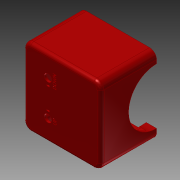
# Autodesk Inventor part: Durometer_Electronics_Enclosure_Lid
Saved by Autodesk Inventor 2015 (Build 190159000, 159)
## iProperties
Created: 2015-01-04
Part Number: Durometer_Electronics_Enclosure_Lid
Material: Generic
Document SubType Name: Modeling
Designer: Drew
Density: 1 g/cm^3
Appearance: Smooth - Red
Author: Drew
Autodesk Inventor part; units mm, degrees
ref_plane "YZ Plane" through (0, 0, 0) normal (1, 0, 0) x (0, 1, 0)
ref_plane "XZ Plane" through (0, 0, 0) normal (0, 1, 0) x (-1, 0, 0)
ref_plane "XY Plane" through (0, 0, 0) normal (0, 0, 1) x (1, 0, 0)
sketch "Sketch1" plane through (0, 0, 0) normal (0, 0, 1) x (1, 0, 0)
  line L0 (28.575, -34.925) -> (-28.575, -34.925)
  line L1 (-34.925, -28.575) -> (-34.925, 28.575)
  line L2 (-28.575, 34.925) -> (28.575, 34.925)
  line L3 (34.925, 28.575) -> (34.925, -28.575)
  line L4 (34.925, -34.925) -> (-34.925, 34.925) construction
  line L5 (-34.925, -34.925) -> (34.925, 34.925) construction
  arc A0 (-28.575, 34.925) -> (-34.925, 28.575) centre (-28.575, 28.575) ccw
  arc A1 (34.925, 28.575) -> (28.575, 34.925) centre (28.575, 28.575) ccw
  arc A2 (28.575, -34.925) -> (34.925, -28.575) centre (28.575, -28.575) ccw
  arc A3 (-34.925, -28.575) -> (-28.575, -34.925) centre (-28.575, -28.575) ccw
  point P0 (0, 0)
  dimension "d0" = 69.85
  dimension "d1" = 69.85
  dimension "d2" = 6.35
  constraints: 12 end point, 8 point on circle, 8 point on line, 8 tangent, 4 centre point, 3 equal radius, 2 midpoint, 2 parallel, 1 horizontal, 1 perpendicular
  measures "d0" distance of L4.end L5.end
  measures "d1" distance between parallel lines of L0 L2
  measures "d2" radius of A0
extrude "Extrusion1" add sketch "Sketch1" along normal blind 50.8
shell "Shell1" thickness 2.032 removed faces 1 at (9.525, 7.4083, 0)
sketch "Sketch4" plane through (0, 0, 0) normal (0, 0, -1) x (-1, 0, 0)
  arc A0 (-32.893, -28.575) -> (-28.575, -32.893) centre (-28.575, -28.575) ccw projected
  line L0 (-43.2886, 0) -> (36.2185, 0)
  line L1 (0, 45.1294) -> (0, -40.5019)
  line L2 (-28.575, -24.257) -> (-32.893, -24.257)
  line L3 (-24.257, -28.575) -> (-24.257, -32.893)
  line L4 (-24.257, -32.893) -> (-28.575, -32.893)
  line L5 (-32.893, -24.257) -> (-32.893, -28.575)
  arc A1 (-32.893, -28.575) -> (-28.575, -32.893) centre (-28.575, -28.575) ccw
  arc A2 (-24.257, -28.575) -> (-28.575, -24.257) centre (-28.575, -28.575) ccw
  arc A3 (-28.575, 32.893) -> (-32.893, 28.575) centre (-28.575, 28.575) ccw
  line L6 (-28.575, 24.257) -> (-32.893, 24.257)
  line L7 (-24.257, 28.575) -> (-24.257, 32.893)
  line L8 (-24.257, 32.893) -> (-28.575, 32.893)
  line L9 (-32.893, 24.257) -> (-32.893, 28.575)
  arc A4 (-28.575, 32.893) -> (-32.893, 28.575) centre (-28.575, 28.575) ccw
  arc A5 (-28.575, 24.257) -> (-24.257, 28.575) centre (-28.575, 28.575) ccw
  arc A6 (28.575, -32.893) -> (32.893, -28.575) centre (28.575, -28.575) ccw
  line L10 (28.575, -24.257) -> (32.893, -24.257)
  line L11 (24.257, -28.575) -> (24.257, -32.893)
  line L12 (24.257, -32.893) -> (28.575, -32.893)
  line L13 (32.893, -24.257) -> (32.893, -28.575)
  arc A7 (28.575, -32.893) -> (32.893, -28.575) centre (28.575, -28.575) ccw
  arc A8 (28.575, -24.257) -> (24.257, -28.575) centre (28.575, -28.575) ccw
  arc A9 (32.893, 28.575) -> (28.575, 32.893) centre (28.575, 28.575) ccw
  line L14 (28.575, 24.257) -> (32.893, 24.257)
  line L15 (24.257, 28.575) -> (24.257, 32.893)
  line L16 (24.257, 32.893) -> (28.575, 32.893)
  line L17 (32.893, 24.257) -> (32.893, 28.575)
  arc A10 (32.893, 28.575) -> (28.575, 32.893) centre (28.575, 28.575) ccw
  arc A11 (24.257, 28.575) -> (28.575, 24.257) centre (28.575, 28.575) ccw
  circle A12 centre (-28.575, -28.575) radius 1.45
  circle A13 centre (-28.575, 28.575) radius 1.45
  circle A14 centre (28.575, -28.575) radius 1.45
  circle A15 centre (28.575, 28.575) radius 1.45
  point P0 (0, 0)
  dimension "d7" = 4.318
  dimension "d8" = 4.318
  dimension "d11" = 2.9
  constraints: 36 end point, 27 symmetric about line, 22 point on circle, 15 centre point, 5 coincident, 4 tangent, 2 horizontal, 2 point on line, 1 vertical, 12 other
  measures "d7" distance of L2.end L5.end
  measures "d8" distance of L3.start L3.end
  measures "d11" diameter of A12
extrude "Extrusion2" add sketch "Sketch4" against normal up to surface (48.768 mm away)
fillet "Fillet2" radius 3.175 24 edges at (33.0651, 33.0651, 50.8) (0, 34.925, 50.8) (-33.0651, 33.0651, 50.8) (-34.925, 0, 50.8) (-33.0651, -33.0651, 50.8) (0, -34.925, 50.8) (33.0651, -33.0651, 50.8) (34.925, 0, 50.8) (32.893, 0, 48.768) (24.257, -30.734, 48.768) (30.734, -24.257, 48.768) (25.5217, -25.5217, 48.768) (0, -32.893, 48.768) (0, 32.893, 48.768) (30.734, 24.257, 48.768) (24.257, 30.734, 48.768) (25.5217, 25.5217, 48.768) (-30.734, -24.257, 48.768) (-24.257, -30.734, 48.768) (-25.5217, -25.5217, 48.768) (-32.893, 0, 48.768) (-24.257, 30.734, 48.768) (-30.734, 24.257, 48.768) (-25.5217, 25.5217, 48.768)
sketch "Sketch5" plane through (0, 0, 50.8) normal (0, 0, 1) x (1, 0, 0)
  circle A0 centre (-12.7, -15.875) radius 3.429
  line L0 (-50.1018, 0) -> (45.2159, 0)
  line L1 (-12.7, -24.1987) -> (-12.7, -7.4873)
  line L2 (-11.43, -9.144) -> (-13.97, -9.144)
  line L3 (-13.97, -9.144) -> (-13.97, -10.414)
  line L4 (-13.97, -10.414) -> (-11.43, -10.414)
  line L5 (-11.43, -10.414) -> (-11.43, -9.144)
  line L6 (-11.43, -9.144) -> (-13.97, -10.414) construction
  line L7 (-13.97, -9.144) -> (-11.43, -10.414) construction
  circle A1 centre (-12.7, 15.875) radius 3.429
  line L8 (-12.7, 24.1987) -> (-12.7, 7.4873)
  line L9 (-11.43, 9.144) -> (-13.97, 9.144)
  line L10 (-13.97, 9.144) -> (-13.97, 10.414)
  line L11 (-13.97, 10.414) -> (-11.43, 10.414)
  line L12 (-11.43, 10.414) -> (-11.43, 9.144)
  line L13 (-11.43, 9.144) -> (-13.97, 10.414) construction
  line L14 (-13.97, 9.144) -> (-11.43, 10.414) construction
  point P0 (0, 0)
  point P1 (-12.7, -9.779)
  point P2 (-12.7, 9.779)
  dimension "d31" = 6.096
  dimension "d32" = 6.858
  dimension "d33" = 2.54
  dimension "d34" = 1.27
  dimension "d35" = 31.75
  dimension "d36" = 12.7
  constraints: 30 end point, 8 symmetric about line, 4 midpoint, 3 point on line, 2 centre point, 2 horizontal, 2 parallel, 1 perpendicular, 1 vertical, 1 other
  measures "d31" distance of A0.centre point (-12.7, -9.779)
  measures "d32" diameter of A0
  measures "d33" distance of L2.start L2.end
  measures "d34" distance of L2.end L3.end
  measures "d35" diameter of A0.centre L0
  measures "d36" horizontal distance of point (0, 0) A0.centre
extrude "Extrusion3" cut sketch "Sketch5" against normal through all
sketch "Sketch6" plane through (0, 0, 50.8) normal (0, 0, 1) x (1, 0, 0)
  line L0 (-8.0796, -18.1611) -> (-8.0796, -12.998) construction
  line L1 (-8.0796, -12.998) -> (-4.9046, -12.998) construction
  line L2 (-4.9046, -12.998) -> (-4.9046, -18.1611) construction
  line L3 (-4.9046, -18.1611) -> (-8.0796, -18.1611) construction
  line L4 (-8.3173, 9.6901) -> (-8.3173, 22.3271) construction
  line L5 (-8.3173, 22.3271) -> (-5.1423, 22.3271) construction
  line L6 (-5.1423, 22.3271) -> (-5.1423, 9.6901) construction
  line L7 (-5.1423, 9.6901) -> (-8.3173, 9.6901) construction
  line L8 (-18.4562, -15.5796) -> (0.4358, -15.5796)
  line L9 (-19.415, 16.0086) -> (-0.523, 16.0086)
  spline S0 degree 2 poles (-4.9674, -16.7878) (-4.9674, -17.057) (-5.1082, -17.4572) (-5.249, -17.598) knots 0 0 0 1 2 2 2
  spline S1 degree 2 poles (-5.249, -17.598) (-5.4071, -17.7585) (-5.8517, -17.8894) (-6.1777, -17.8894) knots 0 0 0 1 2 2 2
  line L10 (-6.1777, -17.8894) -> (-8.0796, -17.8894)
  line L11 (-8.0796, -17.8894) -> (-8.0796, -17.4843)
  line L12 (-8.0796, -17.4843) -> (-6.1777, -17.4843)
  spline S2 degree 2 poles (-6.1777, -17.4843) (-5.9653, -17.4843) (-5.6788, -17.43) (-5.5627, -17.3534) knots 0 0 0 1 2 2 2
  spline S3 degree 2 poles (-5.5627, -17.3534) (-5.4392, -17.2719) (-5.3132, -16.9903) (-5.3132, -16.7878) knots 0 0 0 1 2 2 2
  spline S4 degree 2 poles (-5.3132, -16.7878) (-5.3132, -16.5976) (-5.4392, -16.3012) (-5.5627, -16.2197) knots 0 0 0 1 2 2 2
  spline S5 degree 2 poles (-5.5627, -16.2197) (-5.6788, -16.1431) (-5.9628, -16.0888) (-6.1678, -16.0888) knots 0 0 0 1 2 2 2
  line L13 (-6.1678, -16.0888) -> (-8.0796, -16.0888)
  line L14 (-8.0796, -16.0888) -> (-8.0796, -15.6837)
  line L15 (-8.0796, -15.6837) -> (-6.1777, -15.6837)
  spline S6 degree 2 poles (-6.1777, -15.6837) (-5.8591, -15.6837) (-5.4046, -15.8121) (-5.249, -15.9752) knots 0 0 0 1 2 2 2
  spline S7 degree 2 poles (-5.249, -15.9752) (-5.1057, -16.1209) (-4.9674, -16.5062) (-4.9674, -16.7878) knots 0 0 0 1 2 2 2
  spline S8 degree 2 poles (-7.1608, -13.1766) (-6.9632, -13.1766) (-6.6075, -13.3174) (-6.484, -13.4434) knots 0 0 0 1 2 2 2
  spline S9 degree 2 poles (-6.484, -13.4434) (-6.3284, -13.6015) (-6.1678, -14.0288) (-6.1678, -14.3548) knots 0 0 0 1 2 2 2
  line L16 (-6.1678, -14.3548) -> (-6.1678, -14.6982)
  line L17 (-6.1678, -14.6982) -> (-5.0316, -14.6982)
  line L18 (-5.0316, -14.6982) -> (-5.0316, -15.1033)
  line L19 (-5.0316, -15.1033) -> (-8.0796, -15.1033)
  line L20 (-8.0796, -15.1033) -> (-8.0796, -14.3375)
  spline S10 degree 2 poles (-8.0796, -14.3375) (-8.0796, -14.0658) (-7.9907, -13.6855) (-7.8894, -13.5397) knots 0 0 0 1 2 2 2
  spline S11 degree 2 poles (-7.8894, -13.5397) (-7.7733, -13.3693) (-7.4152, -13.1766) (-7.1608, -13.1766) knots 0 0 0 1 2 2 2
  spline S12 degree 2 poles (-7.1484, -13.599) (-7.3065, -13.599) (-7.5387, -13.7077) (-7.6128, -13.8188) knots 0 0 0 1 2 2 2
  spline S13 degree 2 poles (-7.6128, -13.8188) (-7.677, -13.9152) (-7.7289, -14.1721) (-7.7289, -14.3622) knots 0 0 0 1 2 2 2
  line L21 (-7.7289, -14.3622) -> (-7.7289, -14.6982)
  line L22 (-7.7289, -14.6982) -> (-6.5136, -14.6982)
  line L23 (-6.5136, -14.6982) -> (-6.5136, -14.4215)
  spline S14 degree 2 poles (-6.5136, -14.4215) (-6.5136, -14.1745) (-6.5927, -13.8707) (-6.6964, -13.7719) knots 0 0 0 1 2 2 2
  spline S15 degree 2 poles (-6.6964, -13.7719) (-6.7878, -13.6805) (-7.0027, -13.599) (-7.1484, -13.599) knots 0 0 0 1 2 2 2
  spline S16 degree 2 poles (-6.7266, 12.4021) (-6.3092, 12.4021) (-5.6374, 12.0637) (-5.4496, 11.7797) knots 0 0 0 1 2 2 2
  spline S17 degree 2 poles (-5.4496, 11.7797) (-5.3039, 11.5475) (-5.2051, 11.0708) (-5.2051, 10.7003) knots 0 0 0 1 2 2 2
  line L24 (-5.2051, 10.7003) -> (-5.2051, 9.9988)
  line L25 (-5.2051, 9.9988) -> (-8.2531, 9.9988)
  line L26 (-8.2531, 9.9988) -> (-8.2531, 10.6929)
  spline S18 degree 2 poles (-8.2531, 10.6929) (-8.2531, 11.1227) (-8.1247, 11.6117) (-8.011, 11.7846) knots 0 0 0 1 2 2 2
  spline S19 degree 2 poles (-8.011, 11.7846) (-7.8159, 12.0786) (-7.1712, 12.4021) (-6.7266, 12.4021) knots 0 0 0 1 2 2 2
  spline S20 degree 2 poles (-6.7316, 11.9798) (-7.0823, 11.9798) (-7.5788, 11.7476) (-7.7196, 11.5179) knots 0 0 0 1 2 2 2
  spline S21 degree 2 poles (-7.7196, 11.5179) (-7.8159, 11.3548) (-7.9024, 10.9868) (-7.9024, 10.7126) knots 0 0 0 1 2 2 2
  line L27 (-7.9024, 10.7126) -> (-7.9024, 10.4039)
  line L28 (-7.9024, 10.4039) -> (-5.5558, 10.4039)
  line L29 (-5.5558, 10.4039) -> (-5.5558, 10.7126)
  spline S22 degree 2 poles (-5.5558, 10.7126) (-5.5558, 10.9819) (-5.6423, 11.3894) (-5.7584, 11.5549) knots 0 0 0 1 2 2 2
  spline S23 degree 2 poles (-5.7584, 11.5549) (-5.9016, 11.7673) (-6.3759, 11.9798) (-6.7316, 11.9798) knots 0 0 0 1 2 2 2
  spline S24 degree 2 poles (-7.9048, 14.9981) (-7.7023, 15.171) (-7.1095, 15.3637) (-6.7291, 15.3637) knots 0 0 0 1 2 2 2
  spline S25 degree 2 poles (-6.7291, 15.3637) (-6.3586, 15.3637) (-5.7584, 15.176) (-5.5558, 14.9981) knots 0 0 0 1 2 2 2
  spline S26 degree 2 poles (-5.5558, 14.9981) (-5.3434, 14.8104) (-5.1409, 14.3139) (-5.1409, 14.0151) knots 0 0 0 1 2 2 2
  spline S27 degree 2 poles (-5.1409, 14.0151) (-5.1409, 13.7063) (-5.3508, 13.2123) (-5.5558, 13.032) knots 0 0 0 1 2 2 2
  spline S28 degree 2 poles (-5.5558, 13.032) (-5.7584, 12.8566) (-6.3537, 12.6689) (-6.7291, 12.6689) knots 0 0 0 1 2 2 2
  spline S29 degree 2 poles (-6.7291, 12.6689) (-7.112, 12.6689) (-7.6949, 12.8591) (-7.9048, 13.0345) knots 0 0 0 1 2 2 2
  spline S30 degree 2 poles (-7.9048, 13.0345) (-8.1074, 13.2123) (-8.3173, 13.7088) (-8.3173, 14.0151) knots 0 0 0 1 2 2 2
  spline S31 degree 2 poles (-8.3173, 14.0151) (-8.3173, 14.3263) (-8.1, 14.8252) (-7.9048, 14.9981) knots 0 0 0 1 2 2 2
  spline S32 degree 2 poles (-6.7291, 14.9413) (-7.0304, 14.9413) (-7.4973, 14.8104) (-7.6504, 14.6918) knots 0 0 0 1 2 2 2
  spline S33 degree 2 poles (-7.6504, 14.6918) (-7.8085, 14.5708) (-7.9666, 14.2299) (-7.9666, 14.0175) knots 0 0 0 1 2 2 2
  spline S34 degree 2 poles (-7.9666, 14.0175) (-7.9666, 13.7977) (-7.8134, 13.4667) (-7.6504, 13.3407) knots 0 0 0 1 2 2 2
  spline S35 degree 2 poles (-7.6504, 13.3407) (-7.4948, 13.2197) (-7.0255, 13.0913) (-6.7291, 13.0913) knots 0 0 0 1 2 2 2
  spline S36 degree 2 poles (-6.7291, 13.0913) (-6.1289, 13.0913) (-5.4916, 13.5951) (-5.4916, 14.0175) knots 0 0 0 1 2 2 2
  spline S37 degree 2 poles (-5.4916, 14.0175) (-5.4916, 14.4399) (-6.1289, 14.9413) (-6.7291, 14.9413) knots 0 0 0 1 2 2 2
  line L30 (-8.2531, 19.2243) -> (-5.2051, 18.4586)
  line L31 (-5.2051, 18.4586) -> (-5.2051, 18.0041)
  line L32 (-5.2051, 18.0041) -> (-7.7344, 17.3842)
  line L33 (-7.7344, 17.3842) -> (-5.2051, 16.7815)
  line L34 (-5.2051, 16.7815) -> (-5.2051, 16.3319)
  line L35 (-5.2051, 16.3319) -> (-8.2531, 15.5539)
  line L36 (-8.2531, 15.5539) -> (-8.2531, 15.9713)
  line L37 (-8.2531, 15.9713) -> (-5.7263, 16.5839)
  line L38 (-5.7263, 16.5839) -> (-8.2531, 17.1915)
  line L39 (-8.2531, 17.1915) -> (-8.2531, 17.604)
  line L40 (-8.2531, 17.604) -> (-5.6966, 18.2166)
  line L41 (-5.6966, 18.2166) -> (-8.2531, 18.8266)
  line L42 (-8.2531, 18.8266) -> (-8.2531, 19.2243)
  line L43 (-5.2051, 21.7684) -> (-5.2051, 21.314)
  line L44 (-5.2051, 21.314) -> (-7.8332, 19.9653)
  line L45 (-7.8332, 19.9653) -> (-5.2051, 19.9653)
  line L46 (-5.2051, 19.9653) -> (-5.2051, 19.5874)
  line L47 (-5.2051, 19.5874) -> (-8.2531, 19.5874)
  line L48 (-8.2531, 19.5874) -> (-8.2531, 20.1629)
  line L49 (-8.2531, 20.1629) -> (-5.8399, 21.3905)
  line L50 (-5.8399, 21.3905) -> (-8.2531, 21.3905)
  line L51 (-8.2531, 21.3905) -> (-8.2531, 21.7684)
  line L52 (-8.2531, 21.7684) -> (-5.2051, 21.7684)
  point P0 (0, 0)
  point P1 (-8.3173, 16.0086)
  point P2 (-8.0796, -15.5796)
  dimension "d39" = 3.175
  dimension "d40" = 3.175
  dimension "d41" = 5.1631
  dimension "d42" = 12.637
  constraints: 4 end point, 2 horizontal, 2 midpoint, 2 point on line, 4 other
  measures "d39" distance of L2.end L0.start
  measures "d40" distance of L6.end L4.start
  measures "d41" distance of L1.end L2.end
  measures "d42" distance of L5.end L6.end
extrude "Extrusion4" cut sketch "Sketch6" against normal blind 1.27
sketch "Sketch7" plane through (34.925, -28.575, 0) normal (1, 0, 0) x (0, 0, -1)
  line L0 (-78.8961, 28.575) -> (28.5561, 28.575)
  arc A0 (0, 53.975) -> (0, 3.175) centre (0, 28.575) ccw
  line L1 (0, 3.175) -> (0, 53.975)
  line L2 (0, 4.318) -> (0, 52.832) projected
  point P0 (0, 28.575)
  dimension "d45" = 25.4
  constraints: 4 end point, 3 point on line, 2 point on circle, 1 centre point, 1 coincident, 1 horizontal, 1 midpoint
  measures "d45" radius of A0
extrude "Extrusion5" cut sketch "Sketch7" against normal up to next
equation "\"d1\" = d0"
equation "\"d8\" = d7"
equation "\"d40\" = d39"
body "Solid1"
